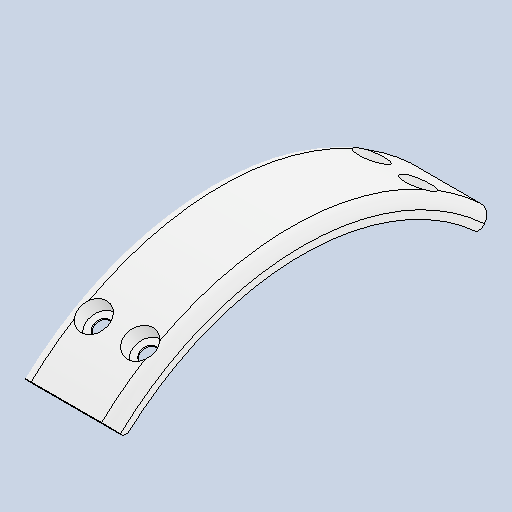
# Autodesk Inventor part: joint3_base_support_fixture
Saved by Autodesk Inventor 2025.3 (Build 293356030, 356C)
## iProperties
Created: 2025-11-25
Part Number: joint3_base_support_fixture
Material: PLA filament
Document SubType Name: Modeling
Designer: MSI
Mass: 14.6457 g
Surface Area: 68.0052 cm^2
Volume: 12.2047 cm^3
Density: 1.2 g/cm^3
Appearance: 일반
Author: MSI
Autodesk Inventor part; units mm, degrees
ref_plane "YZ Plane" through (0, 0, 0) normal (1, 0, 0) x (0, 1, 0)
ref_plane "XZ Plane" through (0, 0, 0) normal (0, 1, 0) x (-1, 0, 0)
ref_plane "XY Plane" through (0, 0, 0) normal (0, 0, 1) x (1, 0, 0)
sketch "스케치1" plane through (0, 0, 0) normal (1, 0, 0) x (0, 1, 0)
  circle A0 centre (0, 0) radius 75
  line L0 (54.8515, 51.1499) -> (0, 0)
  line L1 (0, 0) -> (54.8515, -51.1499)
  line L2 (0, 0) -> (75, 0)
  circle A1 centre (0, 0) radius 70
  point P0 (51.1948, -47.7399)
  point P1 (51.1948, 47.7399)
  dimension "d0" = 150
  dimension "d1" = 43
  dimension "d2" = 43
  dimension "d3" = 5
  constraints: 6 end point, 3 point on circle, 2 centre point, 1 coincident, 1 horizontal
  measures "d0" diameter of A0
  measures "d1" angle of L2 L0
  measures "d2" angle of L2 L1
  measures "d3" radial gap between concentric circles of A0 A1
extrude "돌출1" add sketch "스케치1" along normal mid plane 25 contours L2 A1 L0 A0 | A0 L1 A1 L2
sketch "스케치2" plane through (0, 0, 0) normal (1, 0, 0) x (0, 1, 0)
  arc A0 (54.8515, -51.1499) -> (54.8515, 51.1499) centre (0, 0) ccw projected
  line L0 (64.9519, 37.5) -> (0, 0) construction
  line L1 (0, 0) -> (75, 0) construction
  dimension "d9" = 30
  constraints: 4 end point, 2 point on circle, 1 horizontal
  measures "d9" angle of L1 L0
ref_plane "작업 평면1" through (0, 64.9519, 37.5) normal (0, -0.8660254, -0.5) x (1, 0, 0)
sketch "스케치3" plane through (0, 64.9519, 37.5) normal (0, -0.8660254, -0.5) x (1, 0, 0)
  line L0 (-6.25, 0) -> (6.25, 0) construction
  point P0 (0, 0)
  point P1 (0, 0)
  dimension "d10" = 12.5
  constraints: 3 coincident, 2 end point, 1 horizontal, 1 midpoint
  measures "d10" distance of L0.start L0.end
hole "구멍1" at (-6.25, 64.9519, 37.5) at (6.25, 64.9519, 37.5) direction (0, -0.8660254, -0.5) diameter 4.5 end through all counterbore diameter 8 counterbore depth 4.6 clearance for "Socket Head Cap Screw ISO 4762" size "M4" standard "ISO"
mirror "미러1" about plane through (0, 0, 0) normal (0, 0, 1) of "구멍1"
chamfer "모따기1" distance 1 angle 45 2 edges at (0, 51.1948, 47.7399) (0, 51.1948, -47.7399)
fillet "모깎기1" radius 3 2 edges at (-12.5, 75, 0) (12.5, 75, 0)
equation "\"d2\" = d1"
